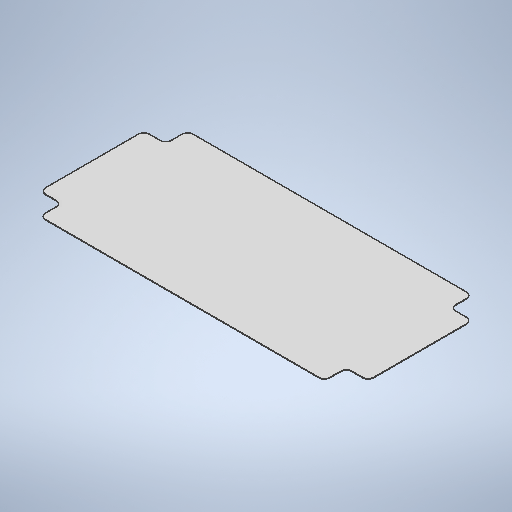
# Autodesk Inventor part: RT_FRM_MC_015_BottomCover
Saved by Autodesk Inventor 2025.3 (Build 293356000, 356)
## iProperties
Created: 2026-06-07
Part Number: RT_FRM_MC_015_BottomCover
Material: Generic
Document SubType Name: Modeling
Designer: louis
Density: 1 g/cm^3
Appearance: Default
Author: louis
Autodesk Inventor part; units mm, degrees
ref_plane "YZ Plane" through (0, 0, 0) normal (1, 0, 0) x (0, 1, 0)
ref_plane "XZ Plane" through (0, 0, 0) normal (0, 1, 0) x (-1, 0, 0)
ref_plane "XY Plane" through (0, 0, 0) normal (0, 0, 1) x (1, 0, 0)
sketch "Sketch1" plane through (0, 0, 0) normal (0, 0, 1) x (1, 0, 0)
  line L0 (-300, -135) -> (300, -135)
  line L1 (300, -135) -> (300, 135)
  line L2 (300, 135) -> (-300, 135)
  line L3 (-300, 135) -> (-300, -135)
  line L4 (-300, -135) -> (300, 135) construction
  line L5 (300, -135) -> (-300, 135) construction
  line L6 (-300, 135) -> (-260, 135)
  line L7 (-260, 135) -> (-260, 95)
  line L8 (-260, 95) -> (-300, 95)
  line L9 (-300, 95) -> (-300, 135)
  line L10 (300, 135) -> (260, 135)
  line L11 (260, 135) -> (260, 95)
  line L12 (260, 95) -> (300, 95)
  line L13 (300, 95) -> (300, 135)
  line L14 (-300, -135) -> (-260, -135)
  line L15 (-260, -135) -> (-260, -95)
  line L16 (-260, -95) -> (-300, -95)
  line L17 (-300, -95) -> (-300, -135)
  line L18 (300, -135) -> (260, -135)
  line L19 (260, -135) -> (260, -95)
  line L20 (260, -95) -> (300, -95)
  line L21 (300, -95) -> (300, -135)
  line L22 (-280, 95) -> (-280, -95) construction
  line L23 (-260, -115) -> (260, -115) construction
  line L24 (280, -95) -> (280, 95) construction
  line L25 (-260, 115) -> (260, 115) construction
  point P0 (0, 0)
  point P1 (300, -95)
  point P2 (300, 95)
  point P3 (-260, 135)
  point P4 (-300, -95)
  dimension "d0" = 600
  dimension "d1" = 270
  dimension "d2" = 40
  dimension "d3" = 40
  dimension "d4" = 40
  dimension "d5" = 40
  dimension "d6" = 40
  dimension "d7" = 40
  dimension "d8" = 40
  dimension "d9" = 40
  constraints: 52 end point, 11 midpoint, 10 parallel, 5 horizontal, 5 perpendicular
  measures "d0" distance of L2.end L1.end
  measures "d1" distance of L1.end L0.end
  measures "d2" distance of L7.end L8.end
  measures "d3" distance of L6.end L7.end
  measures "d4" distance of L12.end L11.end
  measures "d5" distance of L11.end L10.end
  measures "d6" distance of L16.end L15.end
  measures "d7" distance of L19.end L20.end
  measures "d8" distance of L18.end L19.end
  measures "d9" distance of L14.end L15.end
extrude "Extrusion1" add sketch "Sketch1" along normal blind 0.8 contours L15 L16 L3 L8 L7 L2 L11 L12 L1 L20 L19 L0
fillet "Fillet1" radius 10 12 edges at (-300, 95, 0.4) (-260, 95, 0.4) (-260, 135, 0.4) (260, 95, 0.4) (260, 135, 0.4) (300, 95, 0.4) (260, -135, 0.4) (260, -95, 0.4) (300, -95, 0.4) (-260, -95, 0.4) (-260, -135, 0.4) (-300, -95, 0.4)
body "Solid1"
